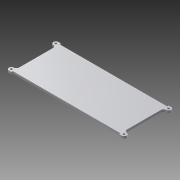
# Autodesk Inventor part: Heatsink
Saved by Autodesk Inventor 2016 (Build 200138000, 138)
## iProperties
Created: 2015-06-09
Part Number: Heatsink
Material: Aluminum 6061
Document SubType Name: Modeling
Designer: Yann
Density: 2.7 g/cm^3
Appearance: Aluminum - Flat
Mass: 133.784 g
Surface Area: 224.248 cm^2
Volume: 49.5496 cm^3
Author: Yann
Autodesk Inventor part; units mm, degrees
ref_plane "YZ Plane" through (0, 0, 0) normal (1, 0, 0) x (0, 1, 0)
ref_plane "XZ Plane" through (0, 0, 0) normal (0, 1, 0) x (-1, 0, 0)
ref_plane "XY Plane" through (0, 0, 0) normal (0, 0, 1) x (1, 0, 0)
sketch "Sketch1" plane through (0, 0, 0) normal (0, 0, 1) x (1, 0, 0)
  line L0 (0, 15198.2615) -> (0, -15198.2615) construction
  line L1 (-114.9467, 0) -> (114.9467, 0) construction
  line L2 (0, -32.5) -> (-75, -32.5)
  line L3 (-75, -32.5) -> (-75, -34.5)
  circle A0 centre (-78.5, -31) radius 1.5
  line L4 (-75, -34.5) -> (-78.5, -34.5)
  arc A1 (-78.7128, -27.5065) -> (-78.5, -34.5) centre (-78.5, -31) ccw
  line L5 (-75, -22.5739) -> (-75, 0)
  line L6 (-78.7128, -27.5065) -> (-75, -27.2803) construction
  line L7 (-75, -27.2803) -> (-75, -22.5739) construction
  spline S0 degree 2 poles (-78.7128, -27.5065) (-75, -27.2803) (-75, -22.5739) knots 1 1 1 2 2 2
  line L8 (0, -32.5) -> (75, -32.5)
  line L9 (75, -32.5) -> (75, -34.5)
  circle A2 centre (78.5, -31) radius 1.5
  line L10 (75, -34.5) -> (78.5, -34.5)
  arc A3 (78.5, -34.5) -> (78.7128, -27.5065) centre (78.5, -31) ccw
  line L11 (75, -22.5739) -> (75, 0)
  line L12 (78.7128, -27.5065) -> (75, -27.2803) construction
  line L13 (75, -27.2803) -> (75, -22.5739) construction
  spline S1 degree 2 poles (78.7128, -27.5065) (75, -27.2803) (75, -22.5739) knots 1 1 1 2 2 2
  line L14 (0, -15198.2615) -> (0, 15198.2615) construction
  line L15 (0, 32.5) -> (-75, 32.5)
  line L16 (-75, 32.5) -> (-75, 34.5)
  circle A4 centre (-78.5, 31) radius 1.5
  line L17 (-75, 34.5) -> (-78.5, 34.5)
  arc A5 (-78.5, 34.5) -> (-78.7128, 27.5065) centre (-78.5, 31) ccw
  line L18 (-75, 22.5739) -> (-75, 0)
  line L19 (-78.7128, 27.5065) -> (-75, 27.2803) construction
  line L20 (-75, 27.2803) -> (-75, 22.5739) construction
  spline S2 degree 2 poles (-78.7128, 27.5065) (-75, 27.2803) (-75, 22.5739) knots 1 1 1 2 2 2
  line L21 (0, 32.5) -> (75, 32.5)
  line L22 (75, 32.5) -> (75, 34.5)
  circle A6 centre (78.5, 31) radius 1.5
  line L23 (75, 34.5) -> (78.5, 34.5)
  arc A7 (78.7128, 27.5065) -> (78.5, 34.5) centre (78.5, 31) ccw
  line L24 (75, 22.5739) -> (75, 0)
  line L25 (78.7128, 27.5065) -> (75, 27.2803) construction
  spline S3 degree 2 poles (78.7128, 27.5065) (75, 27.2803) (75, 22.5739) knots 1 1 1 2 2 2
  line L26 (75, 27.2803) -> (75, 22.5739) construction
  point P0 (0, 0)
  dimension "d0" = 2
  dimension "d1" = 3
  dimension "d3" = 75
  dimension "d4" = 32.5
  dimension "d5" = 3.5
  dimension "d6" = 3.5
  constraints: 34 end point, 28 symmetric about line, 8 centre point, 8 point on circle, 4 coincident, 3 point on line, 2 horizontal, 2 perpendicular, 1 collinear, 1 tangent, 1 vertical, 19 other
  measures "d0" distance of L2.end L3.end
  measures "d1" diameter of A0
  measures "d3" distance of L2.start L2.end
  measures "d4" distance between parallel lines of L1 L2
  measures "d5" distance from line of A1.centre L3
  measures "d6" distance from line of L4 A0.centre
extrude "Extrusion1" add sketch "Sketch1" against normal blind 5
equation "\"d0\" = Cover_Thickness"
equation "\"d3\" = 0.5 * Heatsink_Length"
equation "\"d4\" = 0.5 * Heatsink_Width"
equation "\"d6\" = d5"
equation "\"d7\" = Heatsink_Thickness"
equation "\"Heatsink_Thickness\" = 5"
equation "\"Cover_Thickness\" = 2"
equation "\"Heatsink_Width\" = 65"
equation "\"PowerPCB_Minus_Height\" = 1.2"
equation "\"PowerPCB_Width\" = 63"
equation "\"Interface_Thickness\" = 7"
equation "\"PowerPCB_Thickness\" = 3"
equation "\"PowerPCB_Plus_Height\" = 8"
equation "\"LogicPCB_Width\" = 55"
equation "\"LogicPCB_Thickness\" = 2"
equation "\"LogicPCB_Plus_Height\" = 8"
equation "\"HostPCB_Plus_Height\" = 8"
equation "\"HostPCB_Thickness\" = 1.2"
equation "\"Heatsink_Length\" = 150"
body "Solid1"
